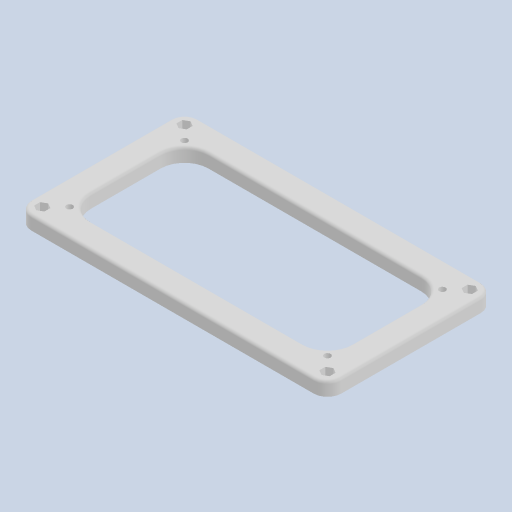
# Autodesk Inventor part: BaseConnector
Saved by Autodesk Inventor 2023 (Build 270158000, 158)
## iProperties
Created: 2024-01-15
Part Number: BaseConnector
Material: Generic
Document SubType Name: Modeling
Designer: Pip
Density: 1 g/cm^3
Appearance: Default
Author: Pip
Autodesk Inventor part; units mm, degrees
ref_plane "YZ Plane" through (0, 0, 0) normal (1, 0, 0) x (0, 1, 0)
ref_plane "XZ Plane" through (0, 0, 0) normal (0, 1, 0) x (-1, 0, 0)
ref_plane "XY Plane" through (0, 0, 0) normal (0, 0, 1) x (1, 0, 0)
sketch "Sketch1" plane through (0, 0, 0) normal (0, 1, 0) x (-1, 0, 0)
  line L0 (95.25, 43) -> (-95.25, 43)
  line L1 (-95.25, 43) -> (-95.25, -43)
  line L2 (-95.25, -43) -> (95.25, -43)
  line L3 (95.25, -43) -> (95.25, 43)
  line L4 (-113.25, 61) -> (113.25, 61)
  line L5 (113.25, 61) -> (113.25, -61)
  line L6 (113.25, -61) -> (-113.25, -61)
  line L7 (-113.25, -61) -> (-113.25, 61)
  line L8 (103.75, -52.25) -> (-103.75, -52.25)
  line L9 (-103.75, -52.25) -> (-103.75, 52.25)
  line L10 (-103.75, 52.25) -> (103.75, 52.25)
  line L11 (103.75, 52.25) -> (103.75, -52.25)
  line L12 (-108.75, -57.25) -> (108.75, -57.25)
  line L13 (108.75, -57.25) -> (108.75, 57.25)
  line L14 (108.75, 57.25) -> (-108.75, 57.25)
  line L15 (-108.75, 57.25) -> (-108.75, -57.25)
  line L16 (108.75, -42.25) -> (103.75, -42.25)
  line L17 (93.75, -52.25) -> (93.75, -57.25)
  line L18 (103.75, 42.25) -> (108.75, 42.25)
  line L19 (93.75, 52.25) -> (93.75, 57.25)
  line L20 (-93.75, 52.25) -> (-93.75, 57.25)
  line L21 (-103.75, 42.25) -> (-108.75, 42.25)
  line L22 (-108.75, -42.25) -> (-103.75, -42.25)
  line L23 (-93.75, -52.25) -> (-93.75, -57.25)
  point P0 (0, 0)
  point P1 (106.25, 42.25)
  dimension "d0" = 86
  dimension "d1" = 190.5
  dimension "d2" = 95.25
  dimension "d3" = 43
  dimension "d4" = 18
  dimension "d11" = 104.5
  dimension "d12" = 52.25
  dimension "d13" = 207.5
  dimension "d14" = 103.75
  dimension "d15" = 5
  dimension "d18" = 15
  dimension "d19" = 15
  dimension "d20" = 15
  dimension "d21" = 15
  dimension "d22" = 15
  dimension "d23" = 15
  dimension "d24" = 15
  dimension "d25" = 15
  constraints: 48 end point, 16 point on line, 12 perpendicular, 8 parallel, 2 horizontal, 1 midpoint, 6 other
  measures "d0" distance of L2.end L0.start
  measures "d1" distance of L1.end L2.end
  measures "d2" distance from line of point (0, 0) L3
  measures "d3" distance from line of L2 point (0, 0)
  measures "d4" distance between parallel lines of L0 L4
  measures "d11" distance between parallel lines of L10 L8
  measures "d12" distance from line of point (0, 0) L10
  measures "d13" distance between parallel lines of L9 L11
  measures "d14" distance from line of point (0, 0) L9
  measures "d15" distance between parallel lines of L8 L12
  measures "d18" distance between parallel lines of L12 L16
  measures "d19" distance between parallel lines of L13 L17
  measures "d20" distance from line of L14 point (106.25, 42.25)
  measures "d21" distance between parallel lines of L13 L19
  measures "d22" distance between parallel lines of L15 L20
  measures "d23" distance between parallel lines of L14 L21
  measures "d24" distance between parallel lines of L12 L22
  measures "d25" distance between parallel lines of L15 L23
extrude "Extrusion1" add sketch "Sketch1" along normal blind 10 contours L4 L5 L6 L7 | L11 L16 L13 L12 L17 L8 | L8 L9 L10 L11 | L17 L12 L23 L8 | L11 L18 L13 L16 | L23 L12 L15 L22 L9 L8 | L11 L10 L19 L14 L13 L18 | L22 L15 L21 L9 | L10 L20 L14 L19 | L21 L15 L14 L20 L10 L9
extrude "Extrusion2" cut sketch "Sketch1" along normal blind 6 contours L17 L12 L23 L8 | L11 L18 L13 L16 | L22 L15 L21 L9 | L10 L20 L14 L19
fillet "Fillet1" radius 10 4 edges at (-113.25, 5, -61) (113.25, 5, -61) (113.25, 5, 61) (-113.25, 5, 61)
fillet "Fillet1" radius 2 8 edges at (113.25, 10, 0) (0, 10, 61) (0, 10, -61) (-113.25, 10, 0) (0, 10, 43) (-95.25, 10, 0) (0, 10, -43) (95.25, 10, 0)
fillet "Fillet1" radius 17.5 4 edges at (-95.25, 5, 43) (-95.25, 5, -43) (95.25, 5, -43) (95.25, 5, 43)
fillet "Fillet2" radius 1 48 edges at (-108.75, 3, 42.25) (-106.25, 6, 42.25) (-103.75, 3, 42.25) (-108.75, 3, -42.25) (-108.75, 6, 0) (-103.75, 3, -42.25) (-106.25, 6, -42.25) (-103.75, 6, 0) (93.75, 3, 57.25) (93.75, 6, 54.75) (93.75, 3, 52.25) (-93.75, 3, 57.25) (0, 6, 57.25) (-93.75, 3, 52.25) (-93.75, 6, 54.75) (0, 6, 52.25) (108.75, 3, -42.25) (106.25, 6, -42.25) (103.75, 3, -42.25) (108.75, 3, 42.25) (108.75, 6, 0) (103.75, 3, 42.25) (106.25, 6, 42.25) (103.75, 6, 0) (93.75, 3, -52.25) (93.75, 6, -54.75) (93.75, 3, -57.25) (-93.75, 3, -52.25) (0, 6, -52.25) (-93.75, 3, -57.25) (-93.75, 6, -54.75) (0, 6, -57.25) (93.75, 0, -54.75) (0, 0, -57.25) (-93.75, 0, -54.75) (0, 0, -52.25) (108.75, 0, 0) (106.25, 0, -42.25) (103.75, 0, 0) (106.25, 0, 42.25) (0, 0, 52.25) (93.75, 0, 54.75) (-93.75, 0, 54.75) (0, 0, 57.25) (-108.75, 0, 0) (-106.25, 0, 42.25) (-103.75, 0, 0) (-106.25, 0, -42.25)
sketch "Sketch3" plane through (0, 10, 0) normal (0, 1, 0) x (1, 0, 0)
  line L0 (-100.5, 54.1651) -> (-100.5, 49.8349)
  line L1 (-100.5, 49.8349) -> (-104.25, 47.6699)
  line L2 (-104.25, 47.6699) -> (-108, 49.8349)
  line L3 (-108, 49.8349) -> (-108, 54.1651)
  line L4 (-108, 54.1651) -> (-104.25, 56.3301)
  line L5 (-104.25, 56.3301) -> (-100.5, 54.1651)
  line L6 (0, 85.4) -> (0, -85.4) projected
  circle A0 centre (-104.25, 52) radius 2.4
  point P0 (0, 0)
  point P1 (-108, 52)
  point P2 (-100.5, 52)
  dimension "d35" = 104.25
  dimension "d36" = 52
  dimension "d39" = 4.8
  dimension "d40" = 7.5
  constraints: 12 end point, 2 midpoint, 1 centre point, 1 coincident, 1 parallel, 13 other
  measures "d35" distance from line of L6 point (-104.25, 52)
  measures "d36" vertical distance of point (0, 0) point (-104.25, 52)
  measures "d39" diameter of A0
  measures "d40" distance of point (-108, 52) point (-100.5, 52)
extrude "Extrusion5" cut sketch "Sketch3" against normal blind 6 contours L0 L1 L2 L3 L4 L5 | A0
extrude "Extrusion6" cut sketch "Sketch3" against normal through all contours A0
sketch "Sketch5" plane through (0, 0, 0) normal (0, -1, 0) x (1, 0, 0)
  line L0 (-97.875, 44.0929) -> (-94.25, 46.1858)
  line L1 (-94.25, 46.1858) -> (-90.625, 44.0929)
  line L2 (-90.625, 44.0929) -> (-90.625, 39.9071)
  line L3 (-90.625, 39.9071) -> (-94.25, 37.8142)
  line L4 (-94.25, 37.8142) -> (-97.875, 39.9071)
  line L5 (-97.875, 39.9071) -> (-97.875, 44.0929)
  line L6 (-113.25, -51) -> (-113.25, 51) projected
  circle A0 centre (-94.25, 42) radius 2.4
  point P0 (0, 0)
  dimension "d45" = 7.25
  dimension "d46" = 94.25
  dimension "d47" = 42
  dimension "d48" = 4.8
  constraints: 12 end point, 1 centre point, 1 coincident, 1 parallel, 13 other
  measures "d45" distance between parallel lines of L5 L2
  measures "d46" horizontal distance of point (0, 0) point (-94.25, 42)
  measures "d47" vertical distance of point (0, 0) point (-94.25, 42)
  measures "d48" diameter of A0
extrude "Extrusion8" cut sketch "Sketch5" against normal blind 3.5 contours L0 L1 L2 L3 L4 L5 | A0
extrude "Extrusion9" cut sketch "Sketch5" against normal through all contours A0
mirror "Mirror1" about plane through (0, 0, 0) normal (0, 0, 1) of "Extrusion6", "Extrusion5", "Extrusion8", "Extrusion9"
mirror "Mirror2" about plane through (0, 0, 0) normal (1, 0, 0) of "Mirror1", "Extrusion6", "Extrusion5", "Extrusion8", "Extrusion9"
sketch "Sketch4" plane through (0, 0, 0) normal (0, -1, 0) x (1, 0, 0)
  line L0 (73.767, -72.0329) -> (-132.5939, -72.0329)
  line L1 (-132.5939, -72.0329) -> (-132.5939, 76.4349)
  line L2 (-132.5939, 76.4349) -> (73.767, 76.4349)
  line L3 (73.767, 76.4349) -> (73.767, -72.0329)
  point P0 (0, 0)
  constraints: 8 end point, 2 parallel, 1 horizontal, 1 perpendicular
equation "\"d0\" = HoleSpacingHoriz - MainThickness"
equation "\"d1\" = HoleSpacingVert - MainThickness"
equation "\"d2\" = 0.5 * d1"
equation "\"d3\" = 0.5 * d0"
equation "\"d4\" = MainThickness"
equation "\"d11\" = SolderSpacingHoriz - SolderThickness"
equation "\"d12\" = 0.5 * d11"
equation "\"d13\" = SolderSpacingVert - SolderThickness"
equation "\"d14\" = 0.5 * d13"
equation "\"d15\" = SolderThickness"
equation "\"d18\" = d19"
equation "\"d20\" = d18"
equation "\"d21\" = d19"
equation "\"d22\" = d19"
equation "\"d23\" = d22"
equation "\"d24\" = d23"
equation "\"d25\" = d23"
equation "\"d35\" = 0.5 * HoleSpacingVert"
equation "\"d36\" = 0.5 * HoleSpacingHoriz"
equation "\"d46\" = 0.5 * InnerHoleSpacingVert"
equation "\"d47\" = 0.5 * InnerHoleSpacingHoriz"
equation "\"HoleSpacingHoriz\" = 104"
equation "\"HoleSpacingVert\" = 208.5"
equation "\"MainThickness\" = 18"
equation "\"SolderSpacingHoriz\" = 109.5"
equation "\"SolderSpacingVert\" = 212.5"
equation "\"SolderThickness\" = 5"
equation "\"InnerHoleSpacingHoriz\" = 84"
equation "\"InnerHoleSpacingVert\" = 188.5"
body "Solid1"
